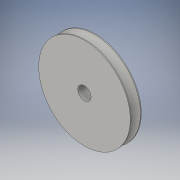
# Autodesk Inventor part: wheel
Saved by Autodesk Inventor 2016 (Build 200138000, 138)
## iProperties
Created: 2019-02-13
Part Number: wheel
Material: Generic
Document SubType Name: Modeling
Designer: reesem783
Density: 1 g/cm^3
Appearance: Default
Author: reesem783
Autodesk Inventor part; units mm, degrees
ref_plane "YZ Plane" through (0, 0, 0) normal (1, 0, 0) x (0, 1, 0)
ref_plane "XZ Plane" through (0, 0, 0) normal (0, 1, 0) x (-1, 0, 0)
ref_plane "XY Plane" through (0, 0, 0) normal (0, 0, 1) x (1, 0, 0)
sketch "Sketch1" plane through (0, 0, 0) normal (1, 0, 0) x (0, 1, 0)
  line L0 (0, 0) -> (0, -3.175)
  line L1 (0, -3.175) -> (-13.208, -3.175)
  line L2 (-13.208, -3.175) -> (-13.208, -2.921)
  line L3 (0, 0) -> (-13.208, 0)
  line L4 (-13.208, 0) -> (-13.208, -0.2327)
  arc A0 (-13.208, -2.921) -> (-13.208, -0.2327) centre (-14.0762, -1.5768) ccw
  dimension "d0" = 3.175
  dimension "d1" = 13.208
  dimension "d4" = 1.6002
  constraints: 10 end point, 3 perpendicular, 2 point on circle, 1 centre point, 1 horizontal, 1 vertical
  measures "d0" distance of L0.start L0.end
  measures "d1" distance of L0.end L1.end
  measures "d4" radius of A0
revolve "Revolution1" add sketch "Sketch1" angle 360 about axis through (0, 0, 0) along (0, 0, -1)
sketch "Sketch2" plane through (0, 0, 0) normal (0, 0, 1) x (1, 0, 0)
  point P0 (0, 0)
  point P1 (0, 0)
  constraints: 1 coincident
hole "Hole1" at (0, 0, 0) direction (0, 0, -1) diameter 3.81 end through all clearance for "Flat Head Machine Screw (82)" size "#6" standard "Ansi Unified Screw Threads"
body "Solid1"
